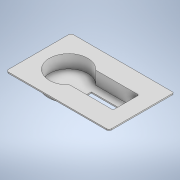
# Autodesk Inventor part: badge
Saved by Autodesk Inventor 2020 (Build 240168000, 168)
## iProperties
Created: 2019-12-22
Part Number: badge
Material: Generic
Document SubType Name: Modeling
Designer: user
Density: 1 g/cm^3
Appearance: Default
Author: user
## iProperties of the stored document _3DPrint.ipt
Created: 2019-12-23
Part Number: _3DPrint
Material: Generic
Document SubType Name: Modeling
Designer: user
Density: 1 g/cm^3
Appearance: Default
Author: user
Autodesk Inventor part; units mm, degrees
ref_plane "YZ Plane" through (0, 0, 0) normal (1, 0, 0) x (0, 1, 0)
ref_plane "XZ Plane" through (0, 0, 0) normal (0, 1, 0) x (-1, 0, 0)
ref_plane "XY Plane" through (0, 0, 0) normal (0, 0, 1) x (1, 0, 0)
sketch "Sketch1" plane through (0, 0, 0) normal (0, 1, 0) x (-1, 0, 0)
  circle A0 centre (-14.3787, -4.818) radius 17
  line L0 (-63.1644, 4.932) -> (-63.1644, -14.568)
  line L1 (-61.1644, -16.568) -> (-26.6644, -16.568)
  line L2 (-26.6644, 6.932) -> (-61.1644, 6.932)
  arc A1 (-63.1644, -14.568) -> (-61.1644, -16.568) centre (-61.1644, -14.568) ccw
  arc A2 (-61.1644, 6.932) -> (-63.1644, 4.932) centre (-61.1644, 4.932) ccw
  line L3 (-29.1287, -0.568) -> (-55.6644, -0.568)
  line L4 (-55.6644, -0.568) -> (-55.6644, -9.068)
  line L5 (-55.6644, -9.068) -> (-29.1287, -9.068)
  line L6 (-29.1287, -9.068) -> (-29.1287, -0.568)
  line L7 (8.6213, 22.172) -> (-72.9787, 22.172)
  line L8 (-73.8987, -31.808) -> (8.6213, -31.808)
  line L9 (10.6213, -29.808) -> (10.6213, 20.172)
  line L10 (-74.9787, 20.172) -> (-74.9787, 4.3466)
  line L11 (-74.9787, -30.728) -> (-74.9787, -14.9025)
  arc A3 (-74.9787, -30.728) -> (-73.8987, -31.808) centre (-73.8987, -30.728) ccw
  arc A4 (-72.9787, 22.172) -> (-74.9787, 20.172) centre (-72.9787, 20.172) ccw
  arc A5 (10.6213, 20.172) -> (8.6213, 22.172) centre (8.6213, 20.172) ccw
  arc A6 (8.6213, -31.808) -> (10.6213, -29.808) centre (8.6213, -29.808) ccw
  line L12 (-74.9787, 4.3466) -> (-74.9787, -14.9025)
  circle A7 centre (-14.3787, -4.818) radius 16
  line L13 (-27.4955, -15.568) -> (-61.1644, -15.568)
  line L14 (-62.1644, -14.568) -> (-62.1644, 4.932)
  arc A8 (-62.1644, -14.568) -> (-61.1644, -15.568) centre (-61.1644, -14.568) ccw
  line L15 (-61.1644, 5.932) -> (-27.5483, 5.932)
  arc A9 (-61.1644, 5.932) -> (-62.1644, 4.932) centre (-61.1644, 4.932) ccw
  line L16 (-26.6644, -16.568) -> (-25.2386, -16.568)
  line L17 (-27.4955, -15.568) -> (-26.2294, -15.568)
  line L18 (-27.5483, 5.932) -> (-26.2294, 5.932)
  line L19 (-26.6644, 6.932) -> (-25.2386, 6.932)
  point P0 (0, 0)
  point P1 (-63.1644, -16.568)
  dimension "d20" = 34
  dimension "d26" = 2
  dimension "d28" = 7.5
  dimension "d32" = 7.5
  dimension "d33" = 7.5
  dimension "d167" = 8.5
  dimension "d171" = 26.5357
  dimension "d177" = 85.6
  dimension "d229" = 32
  dimension "d230" = 1
  dimension "d231" = 1
  dimension "d232" = 1
  dimension "d233" = 1
  dimension "d234" = 1
  dimension "d235" = 1
  dimension "d241" = 53.98
  dimension "d242" = 22.74
  dimension "d243" = 22.74
  constraints: 40 end point, 23 point on circle, 16 tangent, 10 centre point, 6 horizontal, 6 parallel, 3 perpendicular, 3 point on line, 3 vertical, 2 equal radius
  measures "d20" diameter of A0
  measures "d26" radius of A1
  measures "d28" distance between parallel lines of L1 L5
  measures "d32" distance between parallel lines of L3 L2
  measures "d33" distance between parallel lines of L0 L4
  measures "d167" distance between parallel lines of L3 L5
  measures "d171" distance between parallel lines of L4 L6
  measures "d177" distance between parallel lines of L11 L9
  measures "d229" diameter of A7
  measures "d230" radial gap between concentric circles of A0 A7
  measures "d231" distance between parallel lines of L13 L1
  measures "d232" distance between parallel lines of L0 L14
  measures "d233" radius of A8
  measures "d234" distance between parallel lines of L2 L15
  measures "d235" radius of A9
  measures "d241" distance between parallel lines of L8 L7
  measures "d242" distance between parallel lines of L8 L5
  measures "d243" distance between parallel lines of L7 L3
extrude "Extrusion22" add sketch "Sketch1" along normal blind 1
extrude "Extrusion23" add sketch "Sketch1" against normal blind 11 contours A0 L16 A7 L19 | L19 A7 L18 A0 | A0 L15 A9 L14 A8 L13 L1 A1 L0 A2 L2 | A0 L13 L17 A7 L16 | L18 A7 L3 A0 | A0 L3 L4 L5 L13 A8 L14 A9 L15 | A7 L5 L6 L3 | A0 L5 A7 L17 L13 picked at (-18.8787, -4.818)
extrude "Extrusion24" cut sketch "Sketch1" against normal blind 10 contours L18 A7 L3 A0 | A0 L3 L4 L5 L13 A8 L14 A9 L15 | A7 L5 L6 L3 | A0 L5 A7 L17 L13 picked at (-18.8787, -4.818)
extrude "Extrusion25" add sketch "Sketch1" along normal blind 1 contours A0 L16 A7 L19 | L19 A7 L18 A0 | A0 L15 A9 L14 A8 L13 L1 A1 L0 A2 L2 | A0 L13 L17 A7 L16
body "Solid4"
